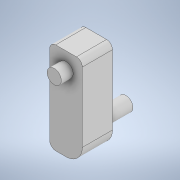
# Autodesk Inventor part: rpi_base_back_gambi
Saved by Autodesk Inventor 2022.1 (Build 261234000, 234)
## iProperties
Created: 2021-07-18
Part Number: rpi_base_back_gambi
Material: Generic
Document SubType Name: Modeling
Designer: dwbertol
Density: 1 g/cm^3
Appearance: Default
Author: dwbertol
## iProperties of the stored document rpi_base_back_3DPrint.ipt
Created: 2021-07-18
Part Number: rpi_base_back_3DPrint
Material: Generic
Document SubType Name: Modeling
Designer: dwbertol
Density: 1 g/cm^3
Appearance: Default
Author: dwbertol
Autodesk Inventor part; units mm, degrees
ref_plane "YZ Plane" through (0, 0, 0) normal (1, 0, 0) x (0, 1, 0)
ref_plane "XZ Plane" through (0, 0, 0) normal (0, 1, 0) x (-1, 0, 0)
ref_plane "XY Plane" through (0, 0, 0) normal (0, 0, 1) x (1, 0, 0)
sketch "Sketch1" plane through (0, 0, 0) normal (0, 0, 1) x (1, 0, 0)
  circle A0 centre (0, 0) radius 1.2
  circle A1 centre (0, 0) radius 2.75
  line L0 (-1.75, 2.75) -> (1.75, 2.75)
  line L1 (2.75, 1.75) -> (2.75, -1.75)
  line L2 (1.75, -2.75) -> (-1.75, -2.75)
  line L3 (-2.75, -1.75) -> (-2.75, 1.75)
  arc A2 (-1.75, 2.75) -> (-2.75, 1.75) centre (-1.75, 1.75) ccw
  arc A3 (2.75, 1.75) -> (1.75, 2.75) centre (1.75, 1.75) ccw
  arc A4 (1.75, -2.75) -> (2.75, -1.75) centre (1.75, -1.75) ccw
  arc A5 (-2.75, -1.75) -> (-1.75, -2.75) centre (-1.75, -1.75) ccw
  line L4 (-2.75, 0) -> (2.75, 0)
  line L5 (2.75, 0) -> (2.75, 11.75)
  line L6 (1.75, 12.75) -> (-1.75, 12.75)
  line L7 (-2.75, 11.75) -> (-2.75, 0)
  circle A6 centre (0, 10) radius 2.75
  circle A7 centre (0, 10) radius 1.2
  arc A8 (-1.75, 12.75) -> (-2.75, 11.75) centre (-1.75, 11.75) ccw
  arc A9 (2.75, 11.75) -> (1.75, 12.75) centre (1.75, 11.75) ccw
  point P0 (-2.75, 0)
  point P1 (0, -2.75)
  point P2 (0, 0)
  point P3 (-2.75, 1.75)
  point P4 (2.75, 0)
  dimension "d0" = 2.4
  dimension "d1" = 5.5
  dimension "d2" = 1
  dimension "d3" = 1
  dimension "d4" = 1
  dimension "d11" = 2.4
  dimension "d12" = 10
  dimension "d13" = 1
  dimension "d14" = 1
  constraints: 19 tangent, 16 end point, 12 point on circle, 10 centre point, 4 parallel, 3 coincident, 2 horizontal, 2 midpoint, 2 perpendicular, 1 collinear, 1 equal radius
  measures "d0" diameter of A0
  measures "d1" diameter of A1
  measures "d2" radius of A2
  measures "d3" radius of A3
  measures "d4" radius of A5
  measures "d11" diameter of A7
  measures "d12" distance of point (0, 0) A6.centre
  measures "d13" radius of A8
  measures "d14" radius of A9
extrude "Extrusion1" add sketch "Sketch1" against normal blind 5 contours L4 A0 | A0 L4
extrude "Extrusion2" add sketch "Sketch1" along normal blind 5.1 contours L4 A0 | L4 A1 A0 | A0 L4 A1 | A0 L4 | A1 L0 A3 L1 | L3 A2 L0 A1 | A1 L2 A5 L3 | L0 A2 L7 A6 L5 A3 | A6 L6 A9 L5 | A6 | L7 A8 L6 A6 | A7
extrude "Extrusion3" add sketch "Sketch1" along normal blind 7.1 contours A7
equation "\"d11\" = d0"
body "Solid1"
